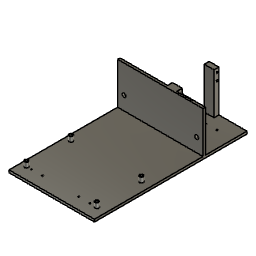
Payload Mount (Autodesk Fusion 360 design; units mm, degrees)
Autodesk Fusion 360 part; units mm, degrees
note: some values were not read from the file. Chosen so that the rebuilt part matches the saved one: which bodies a step acts on. Set by a fixed rule: which sketch regions a step uses.
sketch "Sketch1" plane through (0, 0, 0) normal (0, 0, 1) x (1, 0, 0)
  line L0 (0, 198.4375) -> (111.125, 198.4375)
  line L1 (111.125, 198.4375) -> (111.125, 0)
  line L2 (111.125, 198.4375) -> (89.6938, 198.4375)
  circle A0 centre (75.9063, 180.1813) radius 1
  circle A1 centre (90.1938, 180.1813) radius 1
  circle A2 centre (20.4312, 180.1813) radius 1
  circle A3 centre (34.7188, 180.1813) radius 1
  line L3 (111.125, 198.4375) -> (80.962, 198.4375)
  line L4 (80.962, 198.4375) -> (80.962, 192.0875)
  line L5 (111.125, 0) -> (104.775, 0)
  line L6 (0, 0) -> (111.125, 0)
  circle A4 centre (14.0812, 15.0813) radius 1
  circle A5 centre (28.3687, 15.0813) radius 1
  circle A6 centre (75.4062, 15.0813) radius 1
  circle A7 centre (90.1937, 15.0813) radius 1
  circle A8 centre (7.3495, 15.2875) radius 1.5
  circle A9 centre (99.0125, 15.2875) radius 1.5
  line L7 (80.962, 144.4625) -> (80.962, 150.8125)
  line L8 (80.962, 150.8125) -> (61.912, 150.8125)
  line L9 (61.912, 150.8125) -> (61.912, 144.4625)
  line L10 (80.962, 198.4375) -> (80.962, 192.0875)
  line L11 (80.962, 192.0875) -> (61.912, 192.0875)
  line L12 (61.912, 192.0875) -> (61.912, 198.4375)
  line L13 (0, 0) -> (0, 198.4375)
  line L14 (0, 141.2875) -> (111.125, 141.2875)
  line L15 (61.912, 144.4625) -> (0, 144.4625)
  line L16 (80.962, 144.4625) -> (111.125, 144.4625)
  dimension "d1" = 111.125
  dimension "d2" = 198.4375
  dimension "d3" = 111.125
  dimension "d39" = 14.2875
  dimension "d49" = 6.35
  constraint horizontal L0
  constraint perpendicular L1 L2
  constraint horizontal L3
  constraint vertical L4
  constraint horizontal L5
  constraint coincident L6.start L13.start
  constraint perpendicular L1 L6
  constraint horizontal L8
  constraint perpendicular L7 L8
  constraint perpendicular L11 L12
  constraint perpendicular L0 L13
  constraint coincident L13 L15.end
  constraint perpendicular L13 L15
  constraint coincident L1 L16.end
  constraint perpendicular L1 L16
  measures "d1" distance of L6.start L1.end
  measures "d2" distance of L6.start L0.start
  measures "d3" distance of L0.start L0.end
  measures "d39" distance of A2.centre A3.centre
  measures "d49" distance of L1.end L5.end
extrude "Extrude18" add sketch "Sketch1" along normal blind 3.175 contours L0 L1 L2 L3 L4 L7 L8 L9 L10 L11 L12 L13 L15 L16 makes body 1
extrude "Extrude19" add sketch "Sketch1" along normal blind 3.175 separate body contours L1 L5 L6 L13 L14 makes body 2
extrude "Extrude20" add sketch "Sketch1" along normal blind 57.15 contours L1 L7 L8 L9 L13 L14 L15 L16 bodies 1 2
extrude "Extrude21" add sketch "Sketch1" along normal blind 57.15 contours L0 L4 L10 L11 L12 bodies 1
sketch "Sketch5" plane through (0, 0, 3.175) normal (0, 0, 1) x (-1, 0, 0)
  circle A0 centre (-28.3687, -15.0813) radius 1
  circle A1 centre (-99.0125, -15.2875) radius 1.5
  circle A2 centre (-7.3495, -15.2875) radius 1.5
  circle A3 centre (-90.1937, -15.0813) radius 1
  circle A4 centre (-75.4062, -15.0813) radius 1
  circle A5 centre (-14.0812, -15.0813) radius 1
  line L0 (0, 0) -> (-111.125, 0)
  line L1 (-111.125, 0) -> (-111.125, -141.2875)
  line L2 (-111.125, -141.2875) -> (0, -141.2875)
  line L3 (0, -141.2875) -> (0, 0)
  circle A6 centre (-7.3495, -15.2875) radius 2.5
  circle A7 centre (-99.0125, -15.2875) radius 2.5
  circle A8 centre (-99.0125, -73.2312) radius 1.5
  circle A9 centre (-7.3495, -73.2312) radius 1.5
  dimension "d170" = 1
  dimension "d171" = 1
  dimension "d219" = 3
  measures "d219" diameter of A8
extrude "Extrude24" add sketch "Sketch5" along normal blind 6.35 contours A6 bodies 1
extrude "Extrude25" add sketch "Sketch5" along normal blind 6.35 contours A7 bodies 1
sketch "Sketch6" plane through (61.912, 0, 0) normal (-1, 0, 0) x (0, -1, 0)
  line L0 (-150.8125, 3.175) -> (-144.4625, 3.175)
  line L1 (-144.4625, 3.175) -> (-144.4625, 57.15)
  line L2 (-144.4625, 57.15) -> (-150.8125, 57.15)
  line L3 (-150.8125, 57.15) -> (-150.8125, 3.175)
  circle A0 centre (-196.0563, 52.3875) radius 1.25
  circle A1 centre (-196.0563, 42.8625) radius 1.25
  circle A2 centre (-146.8433, 52.3875) radius 1.25
  circle A3 centre (-146.8433, 42.8625) radius 1.25
extrude "Extrude26" cut sketch "Sketch6" against normal blind 19.05 contours A0 bodies 1
extrude "Extrude27" cut sketch "Sketch6" against normal blind 19.05 contours A1 | A2 | A3 bodies 1
extrude "Extrude28" cut 1 faces at (80.962, 195.4959, 15.9887) along direction (-1, 0, 0) blind 6.35 on bodies 1 bodies 1
extrude "Extrude29" cut 1 faces at (80.962, 147.4039, 15.9887) along direction (-1, 0, 0) blind 6.35 on bodies 1 bodies 1
sketch "Sketch7" plane through (0, 0, 57.15) normal (0, 0, 1) x (-1, 0, 0)
  line L0 (-74.612, -144.4625) -> (-74.612, -150.8125)
  line L1 (-74.612, -150.8125) -> (-61.912, -150.8125)
  line L2 (-61.912, -150.8125) -> (-61.912, -144.4625)
  line L3 (-61.912, -144.4625) -> (0, -144.4625)
  line L4 (0, -144.4625) -> (0, -141.2875)
  line L5 (0, -141.2875) -> (-111.125, -141.2875)
  line L6 (-111.125, -141.2875) -> (-111.125, -144.4625)
  line L7 (-74.612, -144.4625) -> (-74.612, -143.4625)
  line L8 (-74.612, -143.4625) -> (-94.612, -143.4625)
  line L9 (-94.612, -143.4625) -> (-94.612, -144.4625)
  line L10 (-74.612, -144.4625) -> (-94.612, -144.4625)
  dimension "d208" = 20
  constraint coincident L0.start L7.start
  constraint horizontal L8
  constraint perpendicular L9 L10
  measures "d208" distance of L7.end L8.end
extrude "Extrude32" cut sketch "Sketch7" against normal blind 54 bodies 1
extrude "Extrude34" cut 1 faces at (62.1192, 99.547, 3.175) along direction (0, 0, -1) blind 14 on bodies 1 bodies 1 makes body 3 at (100.6667, 17.162, 6.35) makes body 4 at (4.8526, 15.4121, 6.35)
extrude "Extrude35" add sketch "Sketch5" against normal blind 3.175 contours L0 L1 L2 L3 bodies 1 3 4
sketch "Sketch8" plane through (0, 0, 3.175) normal (0, 0, 1) x (-1, 0, 0)
  circle A0 centre (-7.3495, -73.2312) radius 1.5
  circle A1 centre (-99.0125, -15.2875) radius 2.5
  circle A2 centre (-28.3687, -15.0813) radius 1
  circle A3 centre (-75.4062, -15.0813) radius 1
  circle A4 centre (-14.0812, -15.0813) radius 1
  circle A5 centre (-90.1937, -15.0813) radius 1
  circle A6 centre (-7.3495, -15.2875) radius 2.5
  circle A7 centre (-99.0125, -73.2312) radius 1.5
  line L0 (0, -141.2875) -> (0, 0)
  line L1 (0, 0) -> (-111.125, 0)
  line L2 (-111.125, 0) -> (-111.125, -141.2875)
  line L3 (-111.125, -141.2875) -> (0, -141.2875)
  circle A8 centre (-7.3495, -73.2312) radius 2.5
  circle A9 centre (-99.0125, -73.2312) radius 2.5
  dimension "d226" = 1
  dimension "d227" = 1
extrude "Extrude36" add sketch "Sketch8" along normal blind 6.35 contours A8 | A9 bodies 1
sketch "Sketch9" plane through (0, 144.4625, 0) normal (0, 1, 0) x (-1, 0, 0)
  line L0 (-61.912, 3.175) -> (0, 3.175)
  line L1 (0, 3.175) -> (0, 57.15)
  line L2 (0, 57.15) -> (-61.912, 57.15)
  line L3 (-61.912, 57.15) -> (-61.912, 3.175)
  line L4 (-111.125, 57.15) -> (-94.6, 57.15)
  line L5 (-111.125, 57.15) -> (-102.8625, 57.15)
  line L6 (-111.125, 3.175) -> (-111.125, 20.875)
  line L7 (-111.125, 20.875) -> (-102.862, 20.875)
  circle A0 centre (-102.862, 20.875) radius 2.5
  line L8 (0, 3.175) -> (0, 20.875)
  line L9 (0, 20.875) -> (-8.263, 20.875)
  circle A1 centre (-8.263, 20.875) radius 2.5
  dimension "d247" = 17.7
  dimension "d248" = 8.263
  dimension "d249" = 5
  dimension "d250" = 17.7
  dimension "d253" = 5
  constraint horizontal L4
  constraint midpoint L4 L5.end
  constraint horizontal L7
  constraint coincident L7.end A0.centre
  constraint coincident L0.end L1.start
  constraint perpendicular L0 L8
  constraint perpendicular L8 L9
  constraint coincident L9.end A1.centre
  measures "d247" distance of L6.start L6.end
  measures "d248" distance of L6.end L7.end
  measures "d249" diameter of A0
  measures "d250" distance of L0.end L8.end
  measures "d253" diameter of A1
extrude "Extrude40" cut sketch "Sketch9" against normal blind 10 contours A0 | A1 bodies 1
